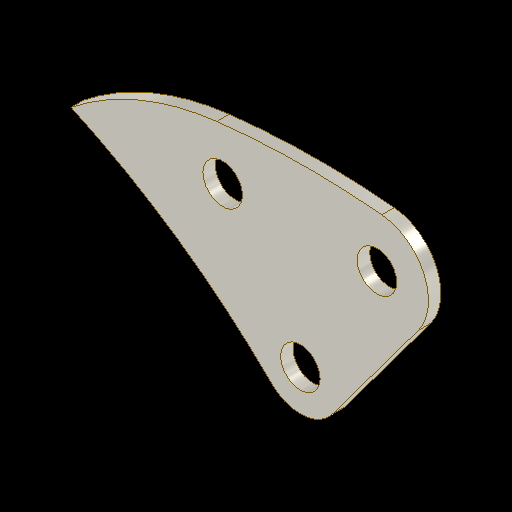
# Autodesk Inventor part: NewTitaniumToothPlate
Saved by Autodesk Inventor 2023 (Build 270158000, 158)
## iProperties
Created: 2022-02-07
Part Number: NewTitaniumToothPlate
Material: Titanium
Document SubType Name: Modeling
Designer: tandu
Density: 4.51 g/cm^3
Appearance: Titanium
Mass: 1.40038 g
Surface Area: 7.22968 cm^2
Volume: 0.310506 cm^3
Author: tandu
Autodesk Inventor part; units mm, degrees
ref_plane "YZ Plane" through (0, 0, 0) normal (1, 0, 0) x (0, 1, 0)
ref_plane "XZ Plane" through (0, 0, 0) normal (0, 1, 0) x (-1, 0, 0)
ref_plane "Work Plane1" through (3.3953, -52.6408, 0) normal (0, 0, 1) x (-0.8454, -0.5341, 0)
sketch "Sketch1" plane through (3.3953, -52.6408, 0) normal (0, 0, 1) x (-0.8454, -0.5341, 0)
  circle A0 centre (-5.4499, -20.2819) radius 4.1275
  circle A1 centre (-5.4499, -20.2819) radius 1.5875 projected
  arc A2 (8.112, -14.595) -> (15.7754, -32.6318) centre (62.4553, -2.1522) ccw
  circle A3 centre (4.9588, -15.317) radius 3.2348
  arc A4 (1.6569, -32.9022) -> (15.7754, -32.6318) centre (7.2596, 43.2761) ccw
  arc A5 (-9.569, -20.0183) -> (1.6569, -32.9022) centre (2.5474, -20.7937) ccw
  line L0 (3.7963, -12.2983) -> (-6.9332, -16.4301)
  circle A6 centre (4.9588, -15.317) radius 1.5875 projected
  circle A7 centre (5.0857, -26.7872) radius 1.5875 projected
  arc A8 (6.7784, 0.693) -> (15.7754, -32.6318) centre (62.4553, -2.1522) ccw projected
  arc A9 (1.6569, -32.9022) -> (15.7754, -32.6318) centre (7.2596, 43.2761) ccw projected
  circle A10 centre (5.0857, -26.7872) radius 4.1275
  arc A11 (-7.9711, -23.5499) -> (3.2933, -30.5052) centre (30.9974, 26.9621) ccw
  arc A12 (3.2933, -30.5052) -> (15.7754, -32.6318) centre (13.2255, -9.9026) ccw
  point P0 (-25.2432, -46.3181)
  point P1 (7.5542, -14.5442)
  point P2 (16.6239, -32.0198)
  dimension "d7" = 2.54
  constraints: 16 point on circle, 8 tangent, 7 centre point, 3 coincident, 2 concentric, 2 end point, 5 other
  measures "d7" radial gap between concentric circles of A1 A0
extrude "Extrusion1" add sketch "Sketch1" along normal blind 1 contours A0 | A10 | A0 L0 A3 A2 A12 A11 | A3
body "Solid1"
